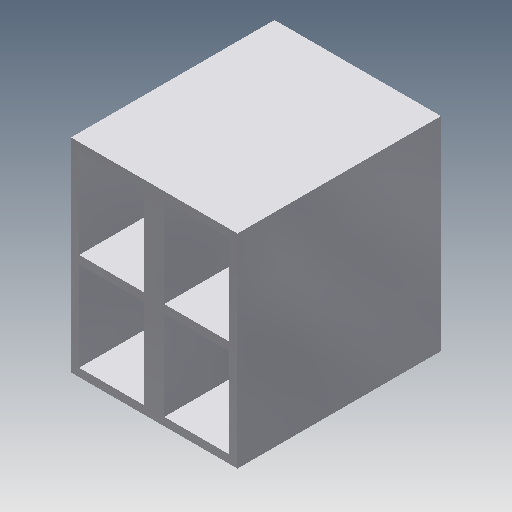
# Autodesk Inventor part: Power Supply Header 2
Saved by Autodesk Inventor 2020 (Build 240152000, 152)
## iProperties
Created: 2005-12-05
Part Number: Power Supply Header 2
Document SubType Name: Modeling
Designer: Simon.Ng@autodesk.com
Stock Number: config - power supply connector
Density: 1 g/cm^3
Material: Generic
Mass: 0.43596 g
Surface Area: 9.6688 cm^2
Volume: 0.43596 cm^3
Appearance: Snow
Company: Autodesk Asia Pte. Ltd.
Title: PC Demo
Author: Simon.Ng@autodesk.com
Autodesk Inventor part; units mm, degrees
ref_plane "YZ Plane" through (0, 0, 0) normal (1, 0, 0) x (0, 1, 0)
ref_plane "XZ Plane" through (0, 0, 0) normal (0, 1, 0) x (-1, 0, 0)
sketch "Sketch1" plane through (0, 0, 0) normal (0, 0, 1) x (1, 0, 0)
  line L0 (0, 8) -> (0, -6) projected
  line L1 (-4.9092, 0) -> (6.5456, 0) projected
  line L2 (-4.091, 5) -> (4.091, 5)
  line L3 (4.091, 5) -> (4.091, -5)
  line L4 (4.091, -5) -> (-4.091, -5)
  line L5 (-4.091, -5) -> (-4.091, 5)
  dimension "d0" = 8.182
  dimension "d1" = 10
  constraints: 8 end point, 2 parallel, 1 horizontal, 1 perpendicular, 2 other
  measures "d0" distance of L2.start L2.end
  measures "d1" distance of L4.end L2.start
extrude "Extrusion1" add sketch "Sketch1" along normal blind 10
sketch "Sketch5" plane through (-4.091, -5, 0) normal (0, -1, 0) x (1, 0, 0)
  line L0 (8.182, 10) -> (0, 10)
  line L1 (2.091, 8) -> (6.091, 8)
  line L2 (6.091, 8) -> (6.091, 5)
  line L3 (6.091, 5) -> (2.091, 5)
  line L4 (2.091, 5) -> (2.091, 8)
  point P0 (4.091, 8)
  point P1 (4.091, 10)
  dimension "d20" = 4
  dimension "d21" = 3
  dimension "d22" = 2
  constraints: 10 end point, 2 midpoint, 2 parallel, 1 horizontal, 1 perpendicular, 1 vertical alignment
  measures "d20" distance of L2.end L3.end
  measures "d21" distance of L1.end L2.end
  measures "d22" distance between parallel lines of L0 L1
extrude "Extrusion5" add sketch "Sketch5" along normal blind 1
ref_plane "Work Plane1" through (0, 0, 10) normal (0, 0, 1) x (1, 0, 0)
sketch "Sketch11" plane through (0, 0, 10) normal (0, 0, 1) x (1, 0, 0)
  line L0 (-0.491, -4.6) -> (-3.691, -4.6)
  line L1 (-3.691, -4.6) -> (-3.691, -0.2)
  line L2 (-3.691, -0.2) -> (-0.491, -0.2)
  line L3 (-0.491, -0.2) -> (-0.491, -4.6)
  line L4 (-4.091, -5) -> (-4.091, 5) projected
  line L5 (4.091, -5) -> (-4.091, -5) projected
  dimension "d57" = 0.4
  dimension "d58" = 0.4
  dimension "d59" = 3.2
  dimension "d60" = 4.4
  constraints: 8 end point, 2 parallel, 1 horizontal, 1 perpendicular
  measures "d57" distance between parallel lines of L5 L0
  measures "d58" distance between parallel lines of L4 L1
  measures "d59" distance of L1.end L2.end
  measures "d60" distance of L2.end L0.start
extrude "Extrusion11" cut sketch "Sketch11" against normal blind 7
pattern_linear "Rectangular Pattern3" count 2 spacing 4.182 along (1, 0, 0) count 2 spacing 4.8 along (0, 1, 0) of "Extrusion11"
body "Solid1"
